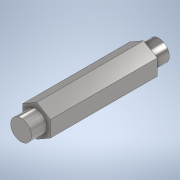
# Autodesk Inventor part: GearShaft
Saved by Autodesk Inventor 2020 (Build 240168000, 168)
## iProperties
Created: 2019-06-01
Part Number: GearShaft
Material: Steel, Alloy
Document SubType Name: Modeling
Designer: Connor
Density: 7.73 g/cm^3
Appearance: Semi-Polished
Author: Connor
Autodesk Inventor part; units mm, degrees
ref_plane "YZ Plane" through (0, 0, 0) normal (1, 0, 0) x (0, 1, 0)
ref_plane "XZ Plane" through (0, 0, 0) normal (0, 1, 0) x (-1, 0, 0)
ref_plane "XY Plane" through (0, 0, 0) normal (0, 0, 1) x (1, 0, 0)
sketch "Sketch1" plane through (0, 0, 0) normal (0, 0, 1) x (1, 0, 0)
  line L0 (0, 7.3323) -> (6.35, 3.6662)
  line L1 (6.35, 3.6662) -> (6.35, -3.6662)
  line L2 (6.35, -3.6662) -> (0, -7.3323)
  line L3 (0, -7.3323) -> (-6.35, -3.6662)
  line L4 (-6.35, -3.6662) -> (-6.35, 3.6662)
  line L5 (-6.35, 3.6662) -> (0, 7.3323)
  point P0 (0, 0)
  point P1 (0, 0)
  dimension "d0" = 12.7
  constraints: 12 end point, 1 coincident, 13 other
  measures "d0" distance between parallel lines of L3 L0
extrude "Extrusion1" add sketch "Sketch1" along normal mid plane 63.5
sketch "Sketch4" plane through (0, 0, 31.75) normal (0, 0, 1) x (1, 0, 0)
  circle A0 centre (0, 0) radius 4.7625
  line L0 (-6.35, 3.6662) -> (-6.35, -3.6662) projected
  line L1 (-6.35, -3.6662) -> (0, -7.3323) projected
  line L2 (0, -7.3323) -> (6.35, -3.6662) projected
  line L3 (6.35, -3.6662) -> (6.35, 3.6662) projected
  line L4 (6.35, 3.6662) -> (0, 7.3323) projected
  line L5 (0, 7.3323) -> (-6.35, 3.6662) projected
  dimension "d7" = 9.525
  constraints: 1 centre point, 1 coincident
  measures "d7" diameter of A0
extrude "Extrusion2" cut sketch "Sketch4" against normal blind 7.1374
mirror "Mirror1" about plane through (0, 0, 0) normal (0, 0, 1) of "Extrusion2"
body "Solid1"
